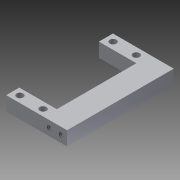
# Autodesk Inventor part: servo_mount
Saved by Autodesk Inventor 2013 (Build 170138000, 138)
## iProperties
Created: 2013-09-17
Part Number: servo_mount
Material: Aluminum 6061
Document SubType Name: Modeling
Designer: Ian
Density: 1 g/cm^3
Author: Ian
Autodesk Inventor part; units mm, degrees
note: some values were not read from the file. Chosen so that the rebuilt part matches the saved one: direction of "Hole1".
ref_plane "YZ Plane" through (0, 0, 0) normal (1, 0, 0) x (0, 1, 0)
ref_plane "XZ Plane" through (0, 0, 0) normal (0, 1, 0) x (-1, 0, 0)
ref_plane "XY Plane" through (0, 0, 0) normal (0, 0, 1) x (1, 0, 0)
sketch "Sketch4" plane through (0, 0, 0) normal (0, 1, 0) x (-1, 0, 0)
  line L0 (-6.35, -28.956) -> (6.35, -28.956)
  line L1 (6.35, -28.956) -> (6.35, 28.956)
  line L2 (6.35, 28.956) -> (-6.35, 28.956)
  line L3 (-6.35, 28.956) -> (-6.35, -28.956)
  line L4 (-6.35, -28.956) -> (6.35, 28.956) construction
  line L5 (6.35, -28.956) -> (-6.35, 28.956) construction
  point P0 (0, 0)
  dimension "d14" = 12.7
  dimension "d15" = 57.912
  constraints: 12 end point, 2 midpoint, 2 parallel, 1 horizontal, 1 perpendicular
  measures "d14" distance of L2.end L1.end
  measures "d15" distance of L1.end L0.end
extrude "Extrusion3" add sketch "Sketch4" along normal blind 7.62
sketch "Sketch5" plane through (-6.35, 0, -28.956) normal (-1, 0, 0) x (0, 0, 1)
  line L0 (0, 0) -> (57.912, 0) projected
  line L1 (57.912, 0) -> (57.912, 7.62) projected
  line L2 (0, 7.62) -> (57.912, 7.62) projected
  line L3 (0, 7.62) -> (7.62, 7.62)
  line L4 (7.62, 7.62) -> (7.62, 0)
  line L5 (7.62, 0) -> (0, 0)
  line L6 (0, 0) -> (0, 7.62)
  line L7 (57.15, 0) -> (50.8, 0)
  line L8 (50.8, 0) -> (50.8, 7.62)
  line L9 (50.8, 7.62) -> (57.912, 7.62)
  line L10 (57.912, 0) -> (57.15, 0)
  point P0 (28.956, 0)
  dimension "d18" = 7.62
  dimension "d21" = 50.8
  constraints: 16 end point, 6 parallel, 3 point on line, 1 collinear, 1 horizontal, 1 perpendicular
  measures "d18" distance of L4.end L5.end
  measures "d21" distance of L7.end L0.start
extrude "Extrusion4" add sketch "Sketch5" along normal blind 20.32 contours L6 L2 L4 L0 | L8 L2 L1 L0
sketch "Sketch6" plane through (0, 7.62, 0) normal (0, 1, 0) x (1, 0, 0)
  line L0 (6.35, -28.956) -> (-26.67, -28.956) projected
  line L1 (6.35, -28.956) -> (6.35, 28.956) projected
  line L2 (-22.7838, 26.9211) -> (-22.7838, -27.5281) construction
  line L3 (-10.1854, 26.9211) -> (-10.1854, -27.5281) construction
  line L4 (-7.0821, 25.146) -> (-30.0582, 25.146) construction
  line L5 (-5.6948, -25.4) -> (-30.0582, -25.4) construction
  point P0 (-26.67, 28.956)
  point P1 (-26.67, 21.336)
  point P2 (-26.67, -21.844)
  point P3 (0, 0)
  point P4 (-22.7838, 25.146)
  point P5 (-10.1854, 25.146)
  point P6 (-10.1854, -25.4)
  point P7 (-22.7838, -25.4)
  dimension "d26" = 3.556
  dimension "d27" = 3.81
  dimension "d28" = 3.8862
  dimension "d29" = 12.5984
  dimension "d30" = 16.4846
  constraints: 8 end point, 8 point on line, 2 parallel, 2 perpendicular
  measures "d26" distance from line of L5 point (-26.67, -21.844)
  measures "d27" vertical distance of point (-26.67, 21.336) L4.end
  measures "d28" horizontal distance of L2.start point (-26.67, 28.956)
  measures "d29" distance of L2.start L3.start
  measures "d30" horizontal distance of L3.start point (-26.67, 28.956)
hole "Hole1" at (-22.7838, 7.62, -25.146) at (-10.1854, 7.62, -25.146) at (-10.1854, 7.62, 25.4) at (-22.7838, 7.62, 25.4) direction (0, -1, 0) diameter 3.6576 end up to surface clearance for "Flat Head Machine Screw (82)" size "#6" standard "Ansi Unified Screw Threads"
sketch "Sketch7" plane through (6.35, 0, 28.956) normal (0, 0, 1) x (1, 0, 0)
  line L0 (0, 0) -> (-33.02, 0) projected
  line L1 (0, 0) -> (0, 7.62) projected
  line L2 (0, 7.62) -> (-33.02, 7.62) projected
  line L3 (-12.7, 0) -> (-12.7, 7.62) projected
  line L4 (-12.7, 7.62) -> (-12.7, 0) projected
  line L5 (-6.5931, 0) -> (-6.5931, 7.62) construction
  line L6 (-12.7, 3.81) -> (-6.5931, 3.81) construction
  line L7 (0, 3.81) -> (-6.5931, 3.81) construction
  point P0 (-6.35, 0)
  point P1 (-9.6465, 3.81)
  point P2 (-3.2965, 3.81)
  dimension "d38" = 6.5931
  constraints: 6 end point, 5 midpoint, 2 point on line, 1 collinear, 1 perpendicular
  measures "d38" distance between parallel lines of L1 L5
hole "Hole2" at (-3.2965, 3.81, 28.956) at (3.0535, 3.81, 28.956) direction (0, 0, -1) diameter 2.6416 depth 12.7 tip angle 118 thread size "6-32 UNC" class "2B" standard "ANSI Unified Screw Threads"
body "Solid2"
